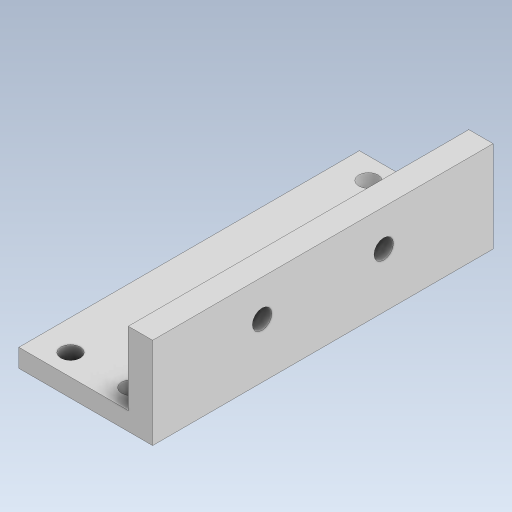
# Autodesk Inventor part: Holder Servo Lifter
Saved by Autodesk Inventor 2023.5 (Build 275446000, 446)
## iProperties
Created: 2025-10-20
Part Number: Holder Servo Lifter
Material: Generic
Document SubType Name: Modeling
Designer: Guntur
Density: 1 g/cm^3
Appearance: Default
Author: Guntur
## iProperties of the stored document Holder Servo Lifter_3DPrint.ipt
Created: 2025-10-20
Part Number: Holder Servo Lifter_3DPrint
Material: Generic
Document SubType Name: Modeling
Designer: Guntur
Density: 1 g/cm^3
Appearance: Default
Author: Guntur
Autodesk Inventor part; units mm, degrees
ref_plane "YZ Plane" through (0, 0, 0) normal (1, 0, 0) x (0, 1, 0)
ref_plane "XZ Plane" through (0, 0, 0) normal (0, 1, 0) x (-1, 0, 0)
ref_plane "XY Plane" through (0, 0, 0) normal (0, 0, 1) x (1, 0, 0)
sketch "Sketch1" plane through (0, 0, 0) normal (0, 1, 0) x (-1, 0, 0)
  line L0 (14.3928, 0) -> (-16, 0) construction
  line L1 (0, 16.4961) -> (0, -25.3301) construction
  circle A0 centre (5, 24.5) radius 1.6
  line L2 (10, 24.5) -> (10, 30)
  line L3 (10, 30) -> (5, 30)
  line L4 (5, 30) -> (0, 30)
  line L5 (0, 30) -> (0, 24.5)
  line L6 (5, 24.5) -> (5, 26.1)
  line L7 (0, 24.5) -> (0, 0)
  line L8 (0, 0) -> (10, 0)
  line L9 (10, 0) -> (10, 24.5)
  circle A1 centre (5, -24.5) radius 1.6
  line L10 (10, -24.5) -> (10, -30)
  line L11 (10, -30) -> (5, -30)
  line L12 (5, -30) -> (0, -30)
  line L13 (0, -30) -> (0, -24.5)
  line L14 (0, -24.5) -> (0, 0)
  line L15 (10, 0) -> (10, -24.5)
  circle A2 centre (-5, 24.5) radius 1.6
  line L16 (-10, 24.5) -> (-10, 30)
  line L17 (-10, 30) -> (-5, 30)
  line L18 (-5, 30) -> (0, 30)
  line L19 (-10, 0) -> (-10, 24.5)
  circle A3 centre (-5, -24.5) radius 1.6
  line L20 (-10, -24.5) -> (-10, -30)
  line L21 (-10, -30) -> (-5, -30)
  line L22 (-5, -30) -> (0, -30)
  line L23 (-10, 0) -> (-10, -24.5)
  line L24 (-10, 30) -> (-8, 30)
  line L25 (-8, 30) -> (-8, -30)
  line L26 (-8, -30) -> (-10, -30)
  line L27 (-10, -30) -> (-10, 30)
  line L28 (10, 30) -> (-10, 30)
  line L29 (-10, 30) -> (-10, 28)
  line L30 (-10, 28) -> (10, 28)
  line L31 (10, 28) -> (10, 30)
  line L32 (-10, -30) -> (10, -30)
  line L33 (10, -30) -> (10, -28)
  line L34 (10, -28) -> (-10, -28)
  line L35 (-10, -28) -> (-10, -30)
  line L36 (-10, -30) -> (-12, -30)
  line L37 (-12, -30) -> (-12, 30)
  line L38 (-12, 30) -> (-10, 30)
  line L39 (-10, 30) -> (-10, -30)
  line L40 (-10, -28) -> (-12, -28)
  line L41 (-10, 28) -> (-12, 28)
  point P0 (5, 27.25)
  point P1 (-8, -28)
  point P2 (-8, 28)
  dimension "d0" = 3.2
  dimension "d2" = 24.5
  dimension "d3" = 5
  dimension "d6" = 2
  constraints: 84 end point, 16 symmetric about line, 10 parallel, 7 perpendicular, 6 horizontal, 5 point on line, 3 centre point, 2 vertical, 1 coincident, 1 vertical alignment, 6 other
  measures "d2" distance from line of L0 point (5, 24.5)
  measures "d3" distance from line of L1 point (5, 24.5)
  measures "d6" distance of L25.end L26.end
extrude "Extrusion1" add sketch "Sketch1" along normal blind 3 contours L9 L8 L7 L5 L30 L2 | L15 L10 L34 L13 L14 L8 | L5 L7 L14 L13 L34 L25 L30 | L25 L34 L20 L23 L19 L16 L30
extrude "Extrusion2" add sketch "Sketch1" along normal blind 15 contours L25 L34 L20 L23 L19 L16 L30 | L16 L19 L23 L20 L40 L37 L41
sketch "Sketch2" plane through (8, 3, 30) normal (-1, 0, 0) x (0, 0, 1)
  line L0 (-58, 12) -> (-2, 12) projected
  line L1 (-30, 12) -> (-30, 0)
  line L2 (-2, 0) -> (-58, 0) projected
  circle A0 centre (-20, 6) radius 1.6
  circle A1 centre (-20, 6) radius 2.75
  circle A2 centre (-40, 6) radius 1.6
  circle A3 centre (-40, 6) radius 2.75
  point P0 (-30, -3)
  point P1 (-60, 12)
  point P2 (0, 12)
  point P3 (0, 0)
  point P4 (-60, 0)
  dimension "d9" = 3.2
  dimension "d10" = 5.5
  dimension "d13" = 10
  constraints: 4 centre point, 2 coincident, 2 end point, 2 midpoint, 2 symmetric about line, 2 other
  measures "d9" diameter of A0
  measures "d10" diameter of A1
  measures "d13" distance from line of L1 A0.centre
extrude "Extrusion3" cut sketch "Sketch2" against normal blind 15 contours A0 | A2
body "Solid1"
